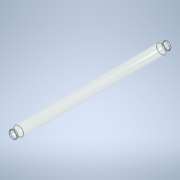
# Autodesk Inventor part: OuterGlassTube
Saved by Autodesk Inventor 2020 (Build 240168000, 168)
## iProperties
Created: 2019-09-29
Part Number: OuterGlassTube
Material: Glass
Document SubType Name: Modeling
Designer: vmiguel
Density: 2.18 g/cm^3
Appearance: Clear
Author: vmiguel
Autodesk Inventor part; units mm, degrees
ref_plane "YZ Plane" through (0, 0, 0) normal (1, 0, 0) x (0, 1, 0)
ref_plane "XZ Plane" through (0, 0, 0) normal (0, 1, 0) x (-1, 0, 0)
ref_plane "XY Plane" through (0, 0, 0) normal (0, 0, 1) x (1, 0, 0)
sketch "Sketch1" plane through (0, 0, 0) normal (0, 0, 1) x (1, 0, 0)
  circle A0 centre (0, 0) radius 15
  circle A1 centre (0, 0) radius 17
  dimension "d0" = 30
  dimension "d1" = 2
  constraints: 2 centre point, 1 coincident
  measures "d0" diameter of A0
  measures "d1" radial gap between concentric circles of A0 A1
extrude "Extrusion1" add sketch "Sketch1" against normal mid plane 480
sketch "Sketch2" plane through (0, 0, 0) normal (1, 0, 0) x (0, 1, 0)
  line L0 (15, -240) -> (15, 240) projected
  line L1 (17, 240) -> (17, -240) projected
  line L2 (14, 255) -> (14, 260)
  line L3 (14, 260) -> (12, 260)
  line L4 (12, 260) -> (12, 255)
  line L5 (17, 240) -> (-17, 240) projected
  line L6 (14, 255) -> (17, 240)
  line L7 (12, 255) -> (15, 240)
  line L8 (0, 0) -> (0, 22.4237)
  dimension "d4" = 2
  dimension "d5" = 2
  dimension "d8" = 12
  dimension "d10" = 5
  dimension "d13" = 20
  constraints: 12 end point, 2 perpendicular, 2 vertical, 1 parallel, 1 other
  measures "d4" distance between parallel lines of L1 L0
  measures "d5" distance of L2.end L3.end
  measures "d8" distance from line of L4 L8.start
  measures "d10" distance of L2.start L2.end
revolve "Revolution1" add sketch "Sketch2" angle 360 about axis through (0, 0, 0) along (0, 0, 1)
fillet "Fillet2" radius 1 1 edges at (0, -14, 260)
mirror "Mirror1" about plane through (0, 0, 0) normal (0, 0, 1) of "Revolution1", "Fillet2"
equation "\"d5\" = d4"
body "Solid1"
